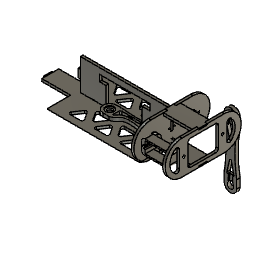
ERA v2.f3d (Autodesk Fusion 360 design; units mm, degrees)
Autodesk Fusion 360 part; units mm, degrees
(part 1 of 2)
sketch "Sketch1" plane through (0, 0, 0) normal (0, 0, 1) x (1, 0, 0)
  line L0 (0, 0) -> (22.8, 0)
  line L1 (22.8, 0) -> (22.8, 28.5)
  line L2 (22.8, 28.5) -> (0, 28.5)
  line L3 (0, 28.5) -> (0, 0)
  dimension "d1" = 22.8
  dimension "d2" = 28.5
  constraint horizontal L0
  constraint vertical L1
  constraint horizontal L2
  constraint vertical L3
  constraint coincident L0.start L3.end
  measures "d1" distance of L0.start L0.end
  measures "d2" distance of L0.start L2.end
sketch "Sketch2" plane through (0, 0, 0) normal (0, 0, 1) x (1, 0, 0)
  line L0 (-2.9, 21.5) -> (-1.5, 21.5)
  line L1 (-1.5, 21.5) -> (-1.5, 19)
  line L2 (-1.5, 19) -> (-2.9, 19)
  line L3 (-2.9, 19) -> (-2.9, 21.5)
  line L4 (0.5, 21.5) -> (1, 21.5)
  line L5 (1, 21.5) -> (1, 23)
  line L6 (1, 23) -> (0.5, 23)
  line L7 (0.5, 23) -> (0.5, 21.5)
  line L8 (-4.7224, 19.0074) -> (27.8871, 19.0074)
  line L9 (27.8871, 19.0074) -> (27.8871, 21.5074)
  line L10 (27.8871, 21.5074) -> (-4.7224, 21.5074)
  line L11 (-4.7224, 21.5074) -> (-4.7224, 19.0074)
  constraint horizontal L0
  constraint vertical L1
  constraint horizontal L2
  constraint vertical L3
  constraint horizontal L4
  constraint vertical L5
  constraint horizontal L6
  constraint vertical L7
  constraint horizontal L8
  constraint vertical L9
  constraint horizontal L10
  constraint vertical L11
sketch "Sketch3" plane through (0, 0, 0) normal (0, 0, 1) x (1, 0, 0)
  line L0 (0, 19) -> (18.5, 19)
  line L1 (18.5, 19) -> (18.5, 21)
  line L2 (18.5, 21) -> (0, 21)
  line L3 (0, 21) -> (0, 19)
  constraint horizontal L0
  constraint vertical L1
  constraint horizontal L2
  constraint vertical L3
sketch "Sketch4" plane through (0, 0, 0) normal (0, 0, 1) x (1, 0, 0)
  line L0 (-25, 0) -> (-47.8, 0)
  line L1 (-47.8, 0) -> (-47.8, 12.2)
  line L2 (-47.8, 12.2) -> (-25, 12.2)
  line L3 (-25, 12.2) -> (-25, 0)
  dimension "d3" = 22.8
  dimension "d4" = 12.2
  constraint horizontal L0
  constraint vertical L1
  constraint horizontal L2
  constraint vertical L3
  measures "d3" distance of L0.start L0.end
  measures "d4" distance of L0.start L2.end
extrude "Extrude1" add sketch "Sketch4" along normal blind 19 makes body 1
sketch "Sketch5" plane through (0, 0, 19) normal (0, 0, 1) x (-1, 0, 0)
  line L0 (25, -12.2) -> (47.8, -12.2)
  line L1 (47.8, -12.2) -> (47.8, 0)
  line L2 (47.8, 0) -> (25, 0)
  line L3 (25, 0) -> (25, -12.2)
  line L4 (52.7, 0) -> (20.1, 0)
  line L5 (20.1, 0) -> (20.1, -12.2)
  line L6 (20.1, -12.2) -> (52.7, -12.2)
  line L7 (52.7, -12.2) -> (52.7, 0)
  dimension "d7" = 32.6
  dimension "d8" = 12.2
  constraint horizontal L4
  constraint vertical L5
  constraint horizontal L6
  constraint vertical L7
  measures "d7" distance of L4.start L4.end
  measures "d8" distance of L4.start L6.end
extrude "Extrude2" add sketch "Sketch5" along normal blind 2.5 bodies 1
move_body "Move1" bodies 1 to x (1, 0, 0) y (0, 1, 0) z (0, 0, 1) at (0, 0, -21.5)
extrude "Extrude3" add sketch "Sketch4" along normal blind 1.5 bodies 1
sketch "Sketch6" plane through (0, 0, 1.5) normal (0, 0, 1) x (-1, 0, 0)
  line L0 (25, -12.2) -> (47.8, -12.2)
  line L1 (47.8, -12.2) -> (47.8, 0)
  line L2 (47.8, 0) -> (25, 0)
  line L3 (25, 0) -> (25, -12.2)
  circle A0 centre (31.1, -6.1) radius 6.1
  circle A1 centre (36.95, -6.05) radius 2
  dimension "d13" = 12.2
  dimension "d14" = 4
  measures "d13" diameter of A0
  measures "d14" diameter of A1
extrude "Extrude4" add sketch "Sketch6" along normal blind 5.5 contours A0 A1 | A0 A1 | A0 A1 bodies 1
sketch "Sketch7" plane through (0, 0, 7) normal (0, 0, 1) x (-1, 0, 0)
  arc A0 (36.8803, -8.0488) -> (36.8462, -4.0527) centre (36.95, -6.05) ccw
  arc A1 (36.8462, -4.0527) -> (36.8803, -8.0488) centre (31.1, -6.1) ccw
  circle A2 centre (31.1, -6.1) radius 2.5
  line L0 (31.1013, -8.6) -> (31.3, -8.3)
  line L1 (31.3, -8.3) -> (30.9, -8.3)
  line L2 (30.9, -8.3) -> (31.1013, -8.6)
  line L3 (31.296, -8.3004) -> (31.5477, -8.5596)
  line L4 (31.5477, -8.5596) -> (31.6896, -8.2289)
  line L5 (31.6858, -8.23) -> (31.9797, -8.4401)
  line L6 (31.9797, -8.4401) -> (32.0603, -8.0894)
  line L7 (32.0567, -8.0912) -> (32.3834, -8.2454)
  line L8 (32.3834, -8.2454) -> (32.4001, -7.886)
  line L9 (32.3969, -7.8883) -> (32.7459, -7.9818)
  line L10 (32.7459, -7.9818) -> (32.6981, -7.6252)
  line L11 (32.6953, -7.628) -> (33.0554, -7.6577)
  line L12 (33.0554, -7.6577) -> (32.9447, -7.3153)
  line L13 (32.9425, -7.3186) -> (33.3021, -7.2835)
  line L14 (33.3021, -7.2835) -> (33.1321, -6.9664)
  line L15 (33.1305, -6.97) -> (33.4781, -6.8713)
  line L16 (33.4781, -6.8713) -> (33.2541, -6.5896)
  line L17 (33.2532, -6.5935) -> (33.5776, -6.4343)
  line L18 (33.5776, -6.4343) -> (33.3069, -6.1971)
  line L19 (33.3068, -6.2011) -> (33.5974, -5.9865)
  line L20 (33.5974, -5.9865) -> (33.2888, -5.8015)
  line L21 (33.2893, -5.8054) -> (33.537, -5.5424)
  line L22 (33.537, -5.5424) -> (33.2003, -5.4155)
  line L23 (33.2016, -5.4193) -> (33.3983, -5.1162)
  line L24 (33.3983, -5.1162) -> (33.0444, -5.0514)
  line L25 (33.0462, -5.0549) -> (33.1857, -4.7216)
  line L26 (33.1857, -4.7216) -> (32.8259, -4.7211)
  line L27 (32.8284, -4.7242) -> (32.9061, -4.3714)
  line L28 (32.9061, -4.3714) -> (32.5519, -4.4351)
  line L29 (32.5549, -4.4377) -> (32.5684, -4.0767)
  line L30 (32.5684, -4.0767) -> (32.2313, -4.2026)
  line L31 (32.2347, -4.2046) -> (32.1835, -3.847)
  line L32 (32.1835, -3.847) -> (31.8743, -4.0311)
  line L33 (31.8781, -4.0325) -> (31.7638, -3.6897)
  line L34 (31.7638, -3.6897) -> (31.4925, -3.9261)
  line L35 (31.4964, -3.9268) -> (31.3228, -3.6099)
  line L36 (31.3228, -3.6099) -> (31.098, -3.8909)
  line L37 (31.102, -3.8909) -> (30.8746, -3.6102)
  line L38 (30.8746, -3.6102) -> (30.7036, -3.9268)
  line L39 (30.7075, -3.9261) -> (30.4336, -3.6904)
  line L40 (30.4336, -3.6904) -> (30.3219, -4.0325)
  line L41 (30.3256, -4.0311) -> (30.0141, -3.8482)
  line L42 (30.0141, -3.8482) -> (29.9653, -4.2046)
  line L43 (29.9687, -4.2026) -> (29.6295, -4.0782)
  line L44 (29.6295, -4.0782) -> (29.6451, -4.4377)
  line L45 (29.6481, -4.4351) -> (29.2921, -4.3733)
  line L46 (29.2921, -4.3733) -> (29.3716, -4.7242)
  line L47 (29.3741, -4.7211) -> (29.0128, -4.7239)
  line L48 (29.0128, -4.7239) -> (29.1538, -5.0549)
  line L49 (29.1556, -5.0514) -> (28.8007, -5.1187)
  line L50 (28.8007, -5.1187) -> (28.9984, -5.4193)
  line L51 (28.9997, -5.4155) -> (28.6624, -5.545)
  line L52 (28.6624, -5.545) -> (28.9107, -5.8054)
  line L53 (28.9112, -5.8015) -> (28.6025, -5.9892)
  line L54 (28.6025, -5.9892) -> (28.8932, -6.2011)
  line L55 (28.8931, -6.1971) -> (28.6228, -6.4369)
  line L56 (28.6228, -6.4369) -> (28.9468, -6.5935)
  line L57 (28.9459, -6.5896) -> (28.7228, -6.8738)
  line L58 (28.7228, -6.8738) -> (29.0695, -6.97)
  line L59 (29.0679, -6.9664) -> (28.8991, -7.2858)
  line L60 (28.8991, -7.2858) -> (29.2575, -7.3186)
  line L61 (29.2553, -7.3153) -> (29.1463, -7.6598)
  line L62 (29.1463, -7.6598) -> (29.5047, -7.628)
  line L63 (29.5019, -7.6252) -> (29.4562, -7.9836)
  line L64 (29.4562, -7.9836) -> (29.8031, -7.8883)
  line L65 (29.7999, -7.886) -> (29.8189, -8.2468)
  line L66 (29.8189, -8.2468) -> (30.1433, -8.0912)
  line L67 (30.1397, -8.0894) -> (30.2228, -8.4411)
  line L68 (30.2228, -8.4411) -> (30.5142, -8.23)
  line L69 (30.5104, -8.2289) -> (30.6549, -8.5601)
  line L70 (30.6549, -8.5601) -> (30.904, -8.3004)
  dimension "d17" = 5
  dimension "d19" = 360
  constraint concentric A1 A2
  constraint coincident A2 L0.start
  constraint horizontal L1
  measures "d17" diameter of A2
extrude "Extrude5" add sketch "Sketch7" along normal blind 4 contours L0 L1 L2 L3 L4 L5 L6 L7 L8 L9 L10 L11 L12 L13 L14 L15 L16 L17 L18 L19 L20 L21 L22 L23 L24 L25 L26 L27 L28 L29 L30 L31 L32 L33 L34 L35 L36 L37 L38 L39 L40 L41 L42 L43 L44 L45 L46 L47 L48 L49 L50 L51 L52 L53 L54 L55 L56 L57 L58 L59 L60 L61 L62 L63 L64 L65 L66 L67 L68 L69 L70 | L0 L1 L2 L3 L70 | L0 L1 L3 | L1 L2 L70 bodies 1
move_body "Move2" bodies 1 to x (1, 0, 0) y (0, 1, 0) z (0, 0, 1) at (0, 0, 21.5)
sketch "Sketch8" plane through (0, 0, 0) normal (0, 0, 1) x (1, 0, 0)
  line L0 (0, 0) -> (77.5, 0)
  line L1 (77.5, 0) -> (77.5, 41.5)
  line L2 (77.5, 41.5) -> (0, 41.5)
  line L3 (0, 41.5) -> (0, 0)
  line L4 (0, 0) -> (77.5, 0)
  line L5 (77.5, 0) -> (77.5, 1)
  line L6 (77.5, 1) -> (0, 1)
  line L7 (0, 1) -> (0, 0)
  line L8 (77.5, 0) -> (76.5, 0)
  line L9 (76.5, 0) -> (76.5, 41.5)
  line L10 (76.5, 41.5) -> (77.5, 41.5)
  line L11 (77.5, 41.5) -> (77.5, 0)
  line L12 (0, 41.5) -> (77.5, 41.5)
  line L13 (77.5, 41.5) -> (77.5, 40.5)
  line L14 (77.5, 40.5) -> (0, 40.5)
  line L15 (0, 40.5) -> (0, 41.5)
  line L16 (0, 41.5) -> (1, 41.5)
  line L17 (1, 41.5) -> (1, 0)
  line L18 (1, 0) -> (0, 0)
  line L19 (0, 0) -> (0, 41.5)
  line L20 (0, 22) -> (77.5, 22)
  line L21 (77.5, 22) -> (77.5, 20)
  line L22 (77.5, 20) -> (0, 20)
  line L23 (0, 20) -> (0, 22)
  dimension "d22" = 77.5
  dimension "d23" = 41.5
  dimension "d24" = 1
  dimension "d25" = 1
  dimension "d26" = 1
  dimension "d27" = 1
  dimension "d28" = 41.5
  dimension "d29" = 77.5
  dimension "d30" = 2
  constraint horizontal L0
  constraint vertical L1
  constraint horizontal L2
  constraint vertical L3
  constraint coincident L0.start L3.end
  constraint horizontal L4
  constraint vertical L5
  constraint horizontal L6
  constraint vertical L7
  constraint horizontal L8
  constraint vertical L9
  constraint horizontal L10
  constraint vertical L11
  constraint coincident L2 L9.end
  constraint horizontal L12
  constraint vertical L13
  constraint horizontal L14
  constraint vertical L15
  constraint coincident L11 L13.end
  constraint horizontal L16
  constraint vertical L17
  constraint horizontal L18
  constraint vertical L19
  constraint horizontal L20
  constraint vertical L21
  constraint horizontal L22
  constraint vertical L23
  constraint coincident L19 L20.start
  measures "d22" distance of L0.start L0.end
  measures "d23" distance of L0.start L2.end
  measures "d24" distance of L0.start L6.end
  measures "d25" distance of L0.end L8.end
  measures "d26" distance of L2.end L14.end
  measures "d27" distance of L2.end L16.end
  measures "d28" distance of L2.end L0.start
  measures "d29" distance of L20.start L20.end
  measures "d30" distance of L20.start L22.end
extrude "Extrude6" add sketch "Sketch8" along normal blind 21.5 separate body contours L0 L3 L4 L6 L7 L17 L18 L19 | L3 L6 L17 L19 L22 | L0 L1 L4 L5 L6 L8 L9 L11 | L3 L17 L19 L20 L22 L23 | L1 L6 L9 L11 L22 | L3 L14 L17 L19 L20 | L1 L9 L11 L20 L21 L22 | L2 L3 L12 L14 L15 L16 L17 L19 | L1 L9 L11 L14 L20 | L1 L2 L9 L10 L11 L12 L13 L14 makes body 2 at (0, 27.6667, 14.3333) makes body 3 at (76.5, 13.8333, 14.3333)
extrude "Extrude7" add sketch "Sketch8" along normal blind 10 contours L0 L4 L6 L9 L17 | L9 L17 L20 L22 | L2 L9 L12 L14 L17 bodies 2 3
extrude "Extrude8" add sketch "Sketch8" along normal blind 1 contours L6 L9 L17 L22 | L9 L14 L17 L20 bodies 2
fillet "Fillet1" radius 5 4 edges at (38.75, 40.5, 1) (38.75, 20, 1) (38.75, 1, 1) (38.75, 22, 1) on bodies 2
fillet "Fillet2" radius 5 6 edges at (1, 0.5, 10) (1, 21, 10) (1, 41, 10) (76.5, 41, 10) (76.5, 21, 10) (76.5, 0.5, 10) on bodies 2
move_body "Move3" bodies 1 to x (1, 0, 0) y (0, 0, 1) z (0, -1, 0) at (0, 0, 0)
copy_body "CopyPasteBodies1" bodies 1 makes body 4
move_body "Move4" bodies 4 to x (1, 0, 0) y (0, -1, 0) z (0, 0, -1) at (0, 41.5, 12)
copy_body "CopyPasteBodies2" bodies 4 1 makes body 5 makes body 6
move_body "Move5" bodies 5 6 to x (1, 0, 0) y (0, 1, 0) z (0, 0, 1) at (150, 0, 0)
sketch "Sketch9" plane through (0, 0, 1) normal (0, 0, 1) x (-1, 0, 0)
  line L0 (-1, -6) -> (-76.5, -6)
  line L1 (-76.5, -6) -> (-76.5, -15)
  line L2 (-76.5, -15) -> (-1, -15)
  line L3 (-1, -15) -> (-1, -6)
  line L4 (144.7876, -93.3118) -> (-10.828, -93.3118) construction
  line L5 (-10.828, -93.3118) -> (-10.828, -128.7007) construction
  line L6 (-10.828, -128.7007) -> (144.7876, -128.7007) construction
  line L7 (144.7876, -128.7007) -> (144.7876, -93.3118) construction
move_body "Move6" bodies 1 4 to x (-1, 0, 0) y (0, 1, 0) z (0, 0, -1) at (-75.4, 0, 12)
move_body "Move7" bodies 1 to x (0, 1, 0) y (1, 0, 0) z (0, 0, -1) at (-27.5, 27.5, 12)
move_body "Move8" bodies 4 to x (0, -1, 0) y (-1, 0, 0) z (0, 0, -1) at (14, 14, 12.4)
move_body "Move9" bodies 5 to x (0, 1, 0) y (1, 0, 0) z (0, 0, -1) at (60.6, -60.6, 12)
move_body "Move10" bodies 6 to x (0, -1, 0) y (-1, 0, 0) z (0, 0, -1) at (102.1, 102.1, 12.4)
move_body "Move11" bodies 1 4 to x (1, 0, 0) y (0, 1, 0) z (0, 0, 1) at (25, 0, 0)
move_body "Move12" bodies 5 6 to x (1, 0, 0) y (0, 1, 0) z (0, 0, 1) at (-22, 0, 0)
move_body "Move13" bodies 1 6 to x (1, 0, 0) y (0, 1, 0) z (0, 0, 1) at (0, 16, 0)
move_body "Move14" bodies 4 5 to x (1, 0, 0) y (0, 1, 0) z (0, 0, 1) at (0, -13, 0)
move_body "Move15" bodies 2 to x (1, 0, 0) y (0, 1, 0) z (0, 0, 1) at (0, -1, 0)
move_body "Move16" bodies 1 6 to x (1, 0, 0) y (0, 1, 0) z (0, 0, 1) at (0, -5.8, 0)
move_body "Move17" bodies 4 5 to x (1, 0, 0) y (0, 1, 0) z (0, 0, 1) at (0, 1.3, 0)
copy_body "CopyPasteBodies3" bodies 1 4 5 6 makes body 7 makes body 8 makes body 9 makes body 10
move_body "Move18" bodies 7 8 9 10 to x (1, 0, 0) y (0, 1, 0) z (0, 0, 1) at (0, -130, 0)
move_body "Move19" bodies 7 to x (0, -1, 0) y (1, 0, 0) z (0, 0, 1) at (80, 29.7, 0)
move_body "Move20" bodies 8 to x (0, 1, 0) y (-1, 0, 0) z (0, 0, 1) at (-139.7, 10.3, 0)
move_body "Move21" bodies 10 to x (0, 1, 0) y (-1, 0, 0) z (0, 0, 1) at (-2.7, -47.9, 0)
move_body "Move22" bodies 9 to x (0, -1, 0) y (1, 0, 0) z (0, 0, 1) at (217.3, 87.9, 0)
move_body "Move23" bodies 1 6 8 9 to x (1, 0, 0) y (0, 1, 0) z (0, 0, 1) at (0, -0.8, 0)
move_body "Move24" bodies 4 5 7 10 to x (1, 0, 0) y (0, 1, 0) z (0, 0, 1) at (0, 0.8, 0)
move_body "Move25" bodies 1 6 8 9 to x (1, 0, 0) y (0, 1, 0) z (0, 0, 1) at (0, -4.5, 0)
move_body "Move26" bodies 4 5 7 10 to x (1, 0, 0) y (0, 1, 0) z (0, 0, 1) at (0, 4.5, 0)
move_body "Move27" bodies 2 to x (1, 0, 0) y (0, 1, 0) z (0, 0, 1) at (0, 170, 0)
move_body "Move28" bodies 5 6 10 9 to x (1, 0, 0) y (0, 1, 0) z (0, 0, 1) at (-34.956, 0, 0)
move_body "Move29" bodies 2 to x (0, 1, 0) y (-1, 0, 0) z (0, 0, 1) at (208, -18.75, 0)
move_body "Move30" bodies 5 6 10 9 to x (1, 0, 0) y (0, 1, 0) z (0, 0, 1) at (-6, 0, 0)
move_body "Move31" bodies 5 6 10 9 to x (1, 0, 0) y (0, 1, 0) z (0, 0, 1) at (5.75, 0, 0)
move_body "Move32" bodies 2 to x (1, 0, 0) y (0, 1, 0) z (0, 0, 1) at (3, 0, 0)
sketch "Sketch10" plane through (0, 0, 0) normal (0, 0, 1) x (1, 0, 0)
  line L0 (-80, -30) -> (120, -30)
  line L1 (120, -30) -> (120, 60)
  line L2 (120, 60) -> (-80, 60)
  line L3 (-80, 60) -> (-80, -30)
  dimension "d41" = 200
  dimension "d42" = 90
  constraint horizontal L0
  constraint vertical L1
  constraint horizontal L2
  constraint vertical L3
  measures "d41" distance of L0.start L0.end
  measures "d42" distance of L0.start L2.end
move_body "Move33" bodies 2 9 4 5 6 1 7 10 8 to x (1, 0, 0) y (0, 1, 0) z (0, 0, 1) at (-1, -5, 0)
move_body "Move34" bodies 2 9 4 5 6 1 7 10 8 to x (1, 0, 0) y (0, 1, 0) z (0, 0, 1) at (0, 0, 4)
move_body "Move35" bodies 4 5 to x (1, 0, 0) y (0, 1, 0) z (0, 0, 1) at (0, -10, 0)
move_body "Move36" bodies 1 6 to x (1, 0, 0) y (0, 1, 0) z (0, 0, 1) at (0, 10, 0)
move_body "Move37" bodies 4 1 to x (1, 0, 0) y (0, 1, 0) z (0, 0, 1) at (-3, 0, 0)
move_body "Move38" bodies 5 6 to x (1, 0, 0) y (0, 1, 0) z (0, 0, 1) at (3, 0, 0)
sketch "Sketch11" plane through (0, 0, 4) normal (0, 0, 1) x (-1, 0, 0)
  line L0 (80, -60) -> (80, 30)
  line L1 (80, 30) -> (-120, 30)
  line L2 (-120, 30) -> (-120, -60)
  line L3 (-120, -60) -> (80, -60)
  line L4 (80, -60) -> (-120, -60)
  line L5 (-120, -60) -> (-120, -56)
  line L6 (-120, -56) -> (80, -56)
  line L7 (80, -56) -> (80, -60)
  line L8 (80, -60) -> (76, -60)
  line L9 (76, -60) -> (76, 30)
  line L10 (76, 30) -> (80, 30)
  line L11 (80, 30) -> (80, -60)
  line L12 (80, 30) -> (-120, 30)
  line L13 (-120, 30) -> (-120, 26)
  line L14 (-120, 26) -> (80, 26)
  line L15 (80, 26) -> (80, 30)
  line L16 (-120, -60) -> (-116, -60)
  line L17 (-116, -60) -> (-116, 30)
  line L18 (-116, 30) -> (-120, 30)
  line L19 (-120, 30) -> (-120, -60)
  dimension "d47" = 4
  dimension "d48" = 4
  dimension "d49" = 4
  dimension "d50" = 4
  constraint horizontal L4
  constraint vertical L5
  constraint horizontal L6
  constraint vertical L7
  constraint coincident L0.start L3.end
  constraint horizontal L8
  constraint vertical L9
  constraint horizontal L10
  constraint vertical L11
  constraint horizontal L12
  constraint vertical L13
  constraint horizontal L14
  constraint vertical L15
  constraint horizontal L16
  constraint vertical L17
  constraint horizontal L18
  constraint vertical L19
  measures "d47" distance of L0.start L6.end
  measures "d48" distance of L0.start L8.end
  measures "d49" distance of L0.end L14.end
  measures "d50" distance of L2.end L16.end
sketch "Sketch12" plane through (-25.5, 0, 0) normal (1, 0, 0) x (0, 1, 0)
  line L0 (-13, 4) -> (-13, 16.2)
  line L1 (-13, 16.2) -> (-17.9, 16.2)
  line L2 (-17.9, 16.2) -> (-17.9, 4)
  line L3 (-17.9, 4) -> (-13, 4)
  line L4 (-13.6, 3.4) -> (10.4, 3.4)
  line L5 (10.4, 3.4) -> (10.4, 16.8)
  line L6 (10.4, 16.8) -> (-13.6, 16.8)
  line L7 (-13.6, 16.8) -> (-13.6, 3.4)
  line L8 (-17.9, 1.6) -> (14.7, 1.6)
  line L9 (14.7, 1.6) -> (14.7, 18.6)
  line L10 (14.7, 18.6) -> (-17.9, 18.6)
  line L11 (-17.9, 18.6) -> (-17.9, 1.6)
  circle A0 centre (-15.9807, 10.1) radius 1
  circle A1 centre (13.0442, 10.1) radius 1
  dimension "d58" = 24
  dimension "d59" = 13.4
  dimension "d60" = 32.6
  dimension "d61" = 17
  dimension "d62" = 2
  dimension "d63" = 2
  constraint horizontal L4
  constraint vertical L5
  constraint horizontal L6
  constraint vertical L7
  constraint horizontal L8
  constraint vertical L9
  constraint horizontal L10
  constraint vertical L11
  measures "d58" distance of L4.start L4.end
  measures "d59" distance of L4.start L6.end
  measures "d60" distance of L8.start L8.end
  measures "d61" distance of L8.start L10.end
  measures "d62" diameter of A0
  measures "d63" diameter of A1
extrude "Extrude11" add sketch "Sketch12" along normal blind 10 separate body contours L1 L3 L4 L5 L6 L7 L8 L9 L10 L11 | L1 L2 L3 L7 L11 makes body 11
sketch "Sketch13" plane through (0, 14.7, 0) normal (0, 1, 0) x (-1, 0, 0)
  line L0 (25.5, 1.6) -> (25.5, 18.6)
  line L1 (25.5, 18.6) -> (15.5, 18.6)
  line L2 (15.5, 18.6) -> (15.5, 1.6)
  line L3 (15.5, 1.6) -> (25.5, 1.6)
  line L4 (25.5, 18.6) -> (6.5, 18.6)
  line L5 (6.5, 18.6) -> (6.5, 1.6)
  line L6 (6.5, 1.6) -> (25.5, 1.6)
  line L7 (25.5, 1.6) -> (25.5, 18.6)
  circle A0 centre (12, 10.1) radius 3.5
  line L8 (15.5, 18.6) -> (15.5, 17.6)
  line L9 (15.5, 1.6) -> (15.5, 2.6)
  line L10 (15.5, 17.6) -> (6.5, 14.5586)
  line L11 (15.5, 2.6) -> (6.5, 5.6414)
  dimension "d66" = 19
  dimension "d67" = 17
  dimension "d68" = 7
  dimension "d69" = 1
  dimension "d70" = 1
  dimension "d107" = 9.5
  dimension "d108" = 9.5
  constraint horizontal L4
  constraint vertical L5
  constraint horizontal L6
  constraint vertical L7
  constraint coincident L0.end L1.start
  constraint coincident L1.end L2.start
  constraint coincident L2 L8.end
  constraint coincident L2.end L3.start
  constraint perpendicular L6 L9
  constraint coincident L5 L10.end
  constraint coincident L5 L11.end
  measures "d66" distance of L0.end L4.end
  measures "d67" distance of L0.end L0.start
  measures "d68" diameter of A0
  measures "d69" distance of L1.end L8.end
  measures "d70" distance of L2.end L9.end
  measures "d107" distance of L8.end L10.end
  measures "d108" distance of L9.end L11.end
extrude "Extrude12" add sketch "Sketch13" against normal blind 4.3 contours L2 L5 L10 L11 bodies 11
sketch "Sketch14" plane through (0, 10.4, 0) normal (0, -1, 0) x (1, 0, 0)
  circle A0 centre (-12, 10.1) radius 3.5
  line L0 (-6.5, 5.6414) -> (-6.5, 14.5586)
  line L1 (-15.5, 3.4) -> (-15.5, 2.6)
  line L2 (-15.5, 16.8) -> (-25.5, 16.8)
  line L3 (-25.5, 16.8) -> (-25.5, 3.4)
  line L4 (-25.5, 3.4) -> (-15.5, 3.4)
  line L5 (-25.5146, 12.3255) -> (-25.5146, 7.9255)
  line L6 (-25.5146, 12.3255) -> (-14.0316, 12.95)
  line L7 (-14.0316, 12.95) -> (-14.0316, 7.25)
  line L8 (-14.0316, 7.25) -> (-25.5146, 7.9255)
  line L9 (-15.5, 2.6) -> (-6.5, 5.6414)
  line L10 (-6.5, 14.5586) -> (-15.5, 17.6)
  line L11 (-15.5, 17.6) -> (-15.5, 16.8)
  dimension "d79" = 4.4
  dimension "d81" = 11.5
  dimension "d82" = 5.7
  constraint vertical L5
  constraint coincident A0 L6.end
  measures "d79" distance of L5.start L5.end
  measures "d81" distance of L5.start L6.end
  measures "d82" distance of L6.end L7.end
extrude "Extrude13" cut sketch "Sketch14" against normal blind 2 contours A0 L3 L6 L8 bodies 11
sketch "Sketch15" plane through (0, -17.9, 0) normal (0, -1, 0) x (1, 0, 0)
  line L0 (-15.5, 1.6) -> (-15.5, 18.6)
  line L1 (-25.5, 18.6) -> (-25.5, 1.6)
  circle A0 centre (-12, 10.1) radius 1.5
  line L2 (-15.5, 18.6) -> (-10.5, 18.6) construction
  line L3 (-15.5, 1.6) -> (-10.5, 1.6) construction
  line L4 (-25.5, 1.6) -> (-15.5, 1.6)
  line L5 (-15.5, 18.6) -> (-25.5, 18.6)
  line L6 (-15.5, 18.6) -> (-8.5, 18.6)
  line L7 (-8.5, 18.6) -> (-8.5, 1.6)
  line L8 (-8.5, 1.6) -> (-15.5, 1.6)
  line L9 (-15.5, 1.6) -> (-15.5, 18.6)
  line L10 (-15.5, 18.6) -> (-15.4999, 18.6)
  line L11 (-15.4999, 18.6) -> (-15.4999, 16.6)
  line L12 (-15.4999, 16.6) -> (-15.5, 16.6)
  line L13 (-15.5, 16.6) -> (-15.5, 18.6)
  line L14 (-15.5, 1.6) -> (-15.5, 3.6)
  line L15 (-15.5, 3.6) -> (-8.5, 8.4218)
  line L16 (-15.4999, 16.6) -> (-8.5, 11.778)
  dimension "d86" = 3
  dimension "d97" = 7
  dimension "d98" = 17
  dimension "d99" = 2
  dimension "d100" = 2
  dimension "d101" = 8.5
  dimension "d102" = 8.5
  constraint horizontal L2
  constraint coincident L0.end L2.start
  constraint horizontal L3
  constraint coincident L0.start L3.start
  constraint horizontal L6
  constraint vertical L7
  constraint horizontal L8
  constraint vertical L9
  constraint horizontal L10
  constraint vertical L11
  constraint horizontal L12
  constraint vertical L13
  constraint perpendicular L8 L14
  constraint coincident L7 L15.end
  constraint coincident L7 L16.end
  measures "d86" diameter of A0
  measures "d97" distance of L0.end L6.end
  measures "d98" distance of L0.end L0.start
  measures "d99" distance of L0.end L12.end
  measures "d100" distance of L0.start L14.end
  measures "d101" distance of L14.end L15.end
  measures "d102" distance of L11.end L16.end
extrude "Extrude14" add sketch "Sketch15" against normal blind 4.3 contours L0 L7 L9 L15 L16 bodies 11
fillet "Fillet9" radius 3 2 edges at (-8.5, -15.75, 11.778) (-8.5, -15.75, 8.4218) on bodies 11
fillet "Fillet10" radius 4 4 edges at (-20.5, -17.9, 18.6) (-20.5, 14.7, 18.6) (-20.5, -17.9, 1.6) (-20.5, 14.7, 1.6) on bodies 11
fillet "Fillet11" radius 4 2 edges at (-6.5, 12.55, 14.5586) (-6.5, 12.55, 5.6414) on bodies 11
move_body "Move39" bodies 11 to x (0, 1, 0) y (1, 0, 0) z (0, 0, -1) at (-50.6, 4.1, 20.2)
copy_body "CopyPasteBodies4" bodies 11 makes body 12
move_body "Move40" bodies 12 to x (1, 0, 0) y (0, 1, 0) z (0, 0, 1) at (-40, 0, 0)
copy_body "CopyPasteBodies5" bodies 11 makes body 13
move_body "Move41" bodies 13 to x (1, 0, 0) y (0, 1, 0) z (0, 0, 1) at (-80, 0, 0)
copy_body "CopyPasteBodies6" bodies 11 makes body 14
move_body "Move42" bodies 14 to x (1, 0, 0) y (0, 1, 0) z (0, 0, 1) at (-120, 0, 0)
move_body "Move43" bodies 12 to x (1, 0, 0) y (0, -1, 0) z (0, 0, -1) at (40, 30.1, 20.2)
move_body "Move44" bodies 13 to x (-1, 0, 0) y (0, -1, 0) z (0, 0, 1) at (-40, 30.1, 0)
move_body "Move45" bodies 14 to x (-1, 0, 0) y (0, 1, 0) z (0, 0, -1) at (-80, 0, 20.2)
sketch "Sketch16" plane through (108.5, 0, 0) normal (1, 0, 0) x (0, 1, 0)
  line L0 (-21.4, 5.6) -> (-8.4965, 5.6)
  line L1 (-8.4965, 5.6) -> (-5.6982, 7.5276)
  arc A0 (-5.6982, 7.5276) -> (-4.4, 9.9982) centre (-7.4, 9.9982) ccw
  line L2 (-4.4, 9.9982) -> (-4.4, 10.2017)
  arc A1 (-4.4, 10.2017) -> (-5.6981, 12.6723) centre (-7.4, 10.2017) ccw
  line L3 (-5.6981, 12.6723) -> (-8.4966, 14.6)
  line L4 (-8.4966, 14.6) -> (-21.4, 14.6)
  line L5 (-21.4, 14.6) -> (-21.4, 5.6)
  circle A2 centre (-7.9, 10.1) radius 1.5
  line L6 (-30, 0) -> (60, 0)
  line L7 (60, 0) -> (60, 40)
  line L8 (60, 40) -> (-30, 40)
  line L9 (-30, 40) -> (-30, 0)
  circle A3 centre (-8.0417, 20.0231) radius 1.5
  line L10 (-8.0417, 20.0231) -> (37.9583, 20.0231)
  circle A4 centre (37.9583, 20.0231) radius 1.5
  dimension "d111" = 90
  dimension "d112" = 40
  dimension "d113" = 3
  dimension "d115" = 46
  dimension "d116" = 3
  constraint horizontal L6
  constraint vertical L7
  constraint horizontal L8
  constraint vertical L9
  constraint coincident A3.centre L10.start
  constraint horizontal L10
  constraint coincident L10.end A4.centre
  measures "d111" distance of L6.start L6.end
  measures "d112" distance of L6.start L8.end
  measures "d113" diameter of A3
  measures "d115" distance of A3.centre L10.end
  measures "d116" diameter of A4
extrude "Extrude15" add sketch "Sketch16" along normal blind 3 separate body contours L0 L1 A0 L2 A1 L3 L4 L5 | A2 | L6 L7 L8 L9 makes body 15
fillet "Fillet12" radius 20 4 edges at (110, -30, 40) (110, -30, 0) (110, 60, 0) (110, 60, 40) on bodies 15
sketch "Sketch17" plane through (111.5, 0, 0) normal (1, 0, 0) x (0, 1, 0)
  arc A0 (40, 0) -> (40, 40) centre (40, 20) ccw
  line L0 (40, 40) -> (-10, 40)
  arc A1 (-10, 40) -> (-10, 0) centre (-10, 20) ccw
  line L1 (-10, 0) -> (40, 0)
  circle A2 centre (-8.0417, 20.0231) radius 1.5
  circle A3 centre (37.9583, 20.0231) radius 1.5
  line L2 (-3, 35) -> (33, 35)
  line L3 (33, 35) -> (33, 5)
  line L4 (33, 5) -> (-3, 5)
  line L5 (-3, 5) -> (-3, 35)
  line L6 (-30, 20) -> (-24.3622, 20)
  line L7 (60, 20) -> (52.8569, 20)
  line L8 (43, 35) -> (43, 5)
  line L9 (-13, 35) -> (-13, 5)
  arc A4 (-13, 35) -> (-13, 5) centre (-8.7798, 20) ccw
  arc A5 (43, 5) -> (43, 35) centre (36.5151, 20) ccw
  dimension "d121" = 36
  dimension "d122" = 30
  constraint horizontal L2
  constraint vertical L3
  constraint horizontal L4
  constraint vertical L5
  constraint midpoint A1 L6.start
  constraint horizontal L6
  constraint midpoint A0 L7.start
  constraint perpendicular L2 L8
  constraint vertical L9
  constraint coincident L6.end A4
  constraint coincident L7.end A5
  measures "d121" distance of L2.start L2.end
  measures "d122" distance of L2.start L4.end
extrude "Extrude16" cut sketch "Sketch17" against normal blind 4 contours L2 L3 L4 L5 | L8 A5 | L9 A4 bodies 15
fillet "Fillet13" radius 3 8 edges at (110, 33, 35) (110, -3, 35) (110, 33, 5) (110, -3, 5) (110, -13, 5) (110, -13, 35) (110, 43, 35) (110, 43, 5) on bodies 15
sketch "Sketch18" plane through (0, 0, 40) normal (0, 0, 1) x (-1, 0, 0)
  line L0 (-111.5, -40) -> (-108.5, -40)
  line L1 (-108.5, -40) -> (-108.5, 10)
  line L2 (-111.5, 10) -> (-111.5, -40)
  line L3 (-74.5, -25) -> (-108.5, -25)
  line L4 (-108.5, -25) -> (-108.5, -5)
  line L5 (-108.5, -5) -> (-74.5, -5)
  line L6 (-74.5, -5) -> (-74.5, -25)
  line L7 (-110, 15) -> (-110, -15)
  line L8 (-108.5, -20) -> (-111.5, -20)
  line L9 (-111.5, -20) -> (-111.5, -10)
  line L10 (-111.5, -10) -> (-108.5, -10)
  line L11 (-108.5, -10) -> (-108.5, -20)
  line L12 (-74.5, -15) -> (35.5, -15)
  line L13 (35.5, -15) -> (35.5, -53)
  line L14 (35.5, -53) -> (-74.5, -53)
  line L15 (-74.5, -53) -> (-74.5, -15)
  line L16 (-74.5, -15) -> (35.5, -15)
  line L17 (35.5, -15) -> (35.5, 23)
  line L18 (35.5, 23) -> (-74.5, 23)
  line L19 (-74.5, 23) -> (-74.5, -15)
  line L20 (35.5, -15) -> (69.5, -15)
  line L21 (69.5, -15) -> (69.5, -25)
  line L22 (69.5, -25) -> (35.5, -25)
  line L23 (35.5, -25) -> (35.5, -15)
  line L24 (35.5, -15) -> (69.5, -15)
  line L25 (69.5, -15) -> (69.5, -5)
  line L26 (69.5, -5) -> (35.5, -5)
  line L27 (35.5, -5) -> (35.5, -15)
  line L28 (69.5, -15) -> (72.5, -15)
  line L29 (72.5, -15) -> (72.5, -20)
  line L30 (72.5, -20) -> (69.5, -20)
  line L31 (69.5, -20) -> (69.5, -15)
  line L32 (69.5, -15) -> (72.5, -15)
  line L33 (72.5, -15) -> (72.5, -10)
  line L34 (72.5, -10) -> (69.5, -10)
  line L35 (69.5, -10) -> (69.5, -15)
  line L36 (-108.5, 10) -> (-111.5, 10)
  dimension "d127" = 34
  dimension "d128" = 20
  dimension "d129" = 30
  dimension "d130" = 3
  dimension "d131" = 10
  dimension "d132" = 110
  dimension "d133" = 38
  dimension "d134" = 38
  dimension "d135" = 34
  dimension "d136" = 10
  dimension "d137" = 10
  dimension "d138" = 3
  dimension "d139" = 5
  constraint horizontal L3
  constraint vertical L4
  constraint horizontal L5
  constraint vertical L6
  constraint coincident L1 L3.end
  constraint horizontal L8
  constraint vertical L9
  constraint horizontal L10
  constraint vertical L11
  constraint coincident L1 L8.start
  constraint horizontal L12
  constraint vertical L13
  constraint horizontal L14
  constraint vertical L15
  constraint midpoint L6 L12.start
  constraint horizontal L16
  constraint vertical L17
  constraint horizontal L18
  constraint vertical L19
  constraint horizontal L20
  constraint vertical L21
  constraint horizontal L22
  constraint vertical L23
  constraint horizontal L24
  constraint vertical L25
  constraint horizontal L26
  constraint vertical L27
  constraint horizontal L28
  constraint vertical L29
  constraint horizontal L30
  constraint vertical L31
  constraint horizontal L32
  constraint vertical L33
  constraint horizontal L34
  constraint vertical L35
  measures "d127" distance of L3.start L3.end
  measures "d128" distance of L3.start L5.end
  measures "d129" distance of L7.start L7.end
  measures "d130" distance of L8.start L8.end
  measures "d131" distance of L8.start L10.end
  measures "d132" distance of L12.start L12.end
  measures "d133" distance of L12.start L14.end
  measures "d134" distance of L12.start L18.end
  measures "d135" distance of L12.end L20.end
  measures "d136" distance of L12.end L22.end
  measures "d137" distance of L12.end L26.end
  measures "d138" distance of L20.end L28.end
  measures "d139" distance of L20.end L34.end
extrude "Extrude17" add sketch "Sketch18" along normal blind 3 separate body contours L1 L2 L4 L8 L9 L10 L11 | L1 L3 L4 L5 L6 L11 L15 L19 | L6 L12 L13 L14 L15 L16 L23 | L6 L12 L16 L17 L18 L19 L27 | L13 L20 L21 L22 L23 L24 L31 | L17 L20 L24 L25 L26 L27 L35 | L21 L28 L29 L30 L31 L32 | L25 L28 L32 L33 L34 L35 makes body 16
sketch "Sketch19" plane through (111.5, 0, 0) normal (1, 0, 0) x (0, 1, 0)
  line L0 (33, 32) -> (33, 8)
  line L1 (30, 5) -> (0, 5)
  line L2 (-3, 8) -> (-3, 32)
  line L3 (0, 35) -> (30, 35)
  arc A0 (40, 0) -> (40, 40) centre (40, 20) ccw
  line L4 (40, 40) -> (-10, 40)
  arc A1 (-10, 40) -> (-10, 0) centre (-10, 20) ccw
  line L5 (-10, 0) -> (40, 0)
  circle A2 centre (-8.0417, 20.0231) radius 1.5
  circle A3 centre (37.9583, 20.0231) radius 1.5
  line L6 (15, 40) -> (20, 40)
  line L7 (20, 40) -> (20, 38.5)
  line L8 (20, 38.5) -> (15, 38.5)
  line L9 (15, 38.5) -> (15, 40)
  line L10 (15, 40) -> (10, 40)
  line L11 (15, 38.4991) -> (15, 40)
  line L12 (15, 40) -> (10, 40)
  line L13 (10, 40) -> (10, 38.5)
  line L14 (10, 38.5) -> (15, 38.5)
  line L15 (15, 38.5) -> (15, 40)
  line L16 (10, 0) -> (20, 0)
  line L17 (20, 0) -> (20, 1.5)
  line L18 (20, 1.5) -> (10, 1.5)
  line L19 (10, 1.5) -> (10, 0)
  arc A4 (30, 5) -> (33, 8) centre (30, 8) ccw
  arc A5 (-3, 8) -> (0, 5) centre (0, 8) ccw
  arc A6 (0, 35) -> (-3, 32) centre (0, 32) ccw
  arc A7 (33, 32) -> (30, 35) centre (30, 32) ccw
  line L20 (-13, 30.3046) -> (-13, 9.6954)
  arc A8 (-17.7215, 32.7615) -> (-17.7215, 7.2385) centre (-8.7798, 20) ccw
  line L21 (43, 10.617) -> (43, 29.383)
  arc A9 (48.1328, 8.5072) -> (48.1328, 31.4928) centre (36.5151, 20) ccw
  arc A10 (-17.7215, 7.2385) -> (-13, 9.6954) centre (-16, 9.6954) ccw
  arc A11 (-13, 30.3046) -> (-17.7215, 32.7615) centre (-16, 30.3046) ccw
  arc A12 (48.1328, 31.4928) -> (43, 29.383) centre (46, 29.383) ccw
  arc A13 (43, 10.617) -> (48.1328, 8.5072) centre (46, 10.617) ccw
  dimension "d142" = 1.5
  dimension "d143" = 5
  dimension "d149" = 1.5
  constraint horizontal L6
  constraint vertical L7
  constraint horizontal L8
  constraint vertical L9
  constraint midpoint L4 L6.start
  constraint horizontal L10
  constraint vertical L11
  constraint horizontal L12
  constraint vertical L13
  constraint horizontal L14
  constraint vertical L15
  constraint horizontal L16
  constraint vertical L17
  constraint horizontal L18
  constraint vertical L19
  constraint coincident L5 L16.start
  measures "d142" distance of L6.start L8.end
  measures "d143" distance of L6.start L10.end
  measures "d149" distance of L16.start L18.end
extrude "Extrude18" cut sketch "Sketch19" against normal blind 3 contours L4 L6 L7 L8 L9 L11 L15 | L4 L9 L10 L11 L12 L13 L14 L15 bodies 15
sketch "Sketch20" plane through (111.5, 0, 0) normal (1, 0, 0) x (0, 1, 0)
  line L0 (10, 40) -> (20, 40)
  line L1 (20, 40) -> (20, 43)
  line L2 (20, 43) -> (10, 43)
  line L3 (10, 43) -> (10, 40)
  line L4 (10, 40) -> (20, 40)
  line L5 (20, 40) -> (20, 41.5)
  line L6 (20, 41.5) -> (10, 41.5)
  line L7 (10, 41.5) -> (10, 40)
  dimension "d146" = 1.5
  constraint horizontal L4
  constraint vertical L5
  constraint horizontal L6
  constraint vertical L7
  constraint coincident L0.start L3.end
  measures "d146" distance of L0.start L6.end
extrude "Extrude19" cut sketch "Sketch20" against normal blind 3 contours L0 L1 L3 L4 L5 L6 L7 bodies 16
move_body "Move46" bodies 16 to x (1, 0, 0) y (0, 1, 0) z (0, 0, 1) at (0, 0, -3)
extrude "Extrude20" cut sketch "Sketch19" against normal blind 3 contours L5 L16 L17 L18 L19 bodies 15
move_body "Move47" bodies 16 to x (1, 0, 0) y (0, -1, 0) z (0, 0, -1) at (0, 30, 30)
move_body "Move48" bodies 10 9 13 14 to x (1, 0, 0) y (0, 1, 0) z (0, 0, 1) at (-1, 0, 4.9)
move_body "Move49" bodies 5 6 to x (1, 0, 0) y (0, 1, 0) z (0, 0, 1) at (0, 1, 5)
move_body "Move50" bodies 6 to x (1, 0, 0) y (0, 1, 0) z (0, 0, 1) at (0, -2, -0.2)
sketch "Sketch21" plane through (74.5, 0, 0) normal (1, 0, 0) x (0, 1, 0)
  line L0 (5, -7) -> (-23, -7)
  line L1 (-23, -7) -> (-23, -10)
  line L2 (-23, -10) -> (5, -10)
  line L3 (5, -10) -> (5, -7)
  line L4 (-30, 35) -> (60, 35)
  line L5 (60, 35) -> (60, -5)
  line L6 (60, -5) -> (-30, -5)
  line L7 (-30, -5) -> (-30, 35)
  circle A0 centre (-7.9, 15.1) radius 6.1
  circle A1 centre (37.9049, 15.1047) radius 6.1
  circle A2 centre (-2.0555, 15.1538) radius 2
  circle A3 centre (32.0504, 15.0437) radius 2
  line L8 (-18.9, 21.2) -> (-14.1, 21.2)
  line L9 (-14.1, 21.2) -> (-14.1, 9)
  line L10 (-14.1, 9) -> (-18.9, 9)
  line L11 (-18.9, 9) -> (-18.9, 21.2)
  line L12 (8.9, 9) -> (13.7, 9)
  line L13 (13.7, 9) -> (13.7, 21.2)
  line L14 (13.7, 21.2) -> (8.9, 21.2)
  line L15 (8.9, 21.2) -> (8.9, 9)
  line L16 (16.3, 21.2) -> (21.1, 21.2)
  line L17 (21.1, 21.2) -> (21.1, 9)
  line L18 (21.1, 9) -> (16.3, 9)
  line L19 (16.3, 9) -> (16.3, 21.2)
  line L20 (44.1, 9) -> (48.9, 9)
  line L21 (48.9, 9) -> (48.9, 21.2)
  line L22 (48.9, 21.2) -> (44.1, 21.2)
  line L23 (44.1, 21.2) -> (44.1, 9)
  circle A4 centre (-17, 15) radius 1
  circle A5 centre (12, 15) radius 1
  circle A6 centre (18, 15) radius 1
  circle A7 centre (47, 15) radius 1
  dimension "d152" = 90
  dimension "d153" = 40
  dimension "d154" = 12.2
  dimension "d155" = 12.2
  dimension "d156" = 4
  dimension "d157" = 4
  constraint horizontal L4
  constraint vertical L5
  constraint horizontal L6
  constraint vertical L7
  constraint horizontal L8
  constraint vertical L9
  constraint horizontal L10
  constraint vertical L11
  constraint horizontal L12
  constraint vertical L13
  constraint horizontal L14
  constraint vertical L15
  constraint horizontal L16
  constraint vertical L17
  constraint horizontal L18
  constraint vertical L19
  constraint horizontal L20
  constraint vertical L21
  constraint horizontal L22
  constraint vertical L23
  measures "d152" distance of L4.start L4.end
  measures "d153" distance of L4.start L6.end
  measures "d154" diameter of A0
  measures "d155" diameter of A1
  measures "d156" diameter of A2
  measures "d157" diameter of A3
extrude "Extrude21" add sketch "Sketch21" against normal blind 3 separate body contours L4 L5 L6 L7 makes body 17
fillet "Fillet14" radius 20 4 edges at (73, -30, 35) (73, -30, -5) (73, 60, 35) (73, 60, -5) on bodies 17
extrude "Extrude22" add sketch "Sketch21" against normal blind 6 contours L8 L9 L10 L11 | L12 L13 L14 L15 | L16 L17 L18 L19 | L20 L21 L22 L23 bodies 17
sketch "Sketch22" plane through (71.5, 0, 0) normal (-1, 0, 0) x (0, -1, 0)
  arc A0 (-40, 35) -> (-40, -5) centre (-40, 15) ccw
  line L0 (-40, -5) -> (10, -5)
  arc A1 (10, -5) -> (10, 35) centre (10, 15) ccw
  line L1 (10, 35) -> (-40, 35)
  line L2 (-8.9, 21.2) -> (-8.9, 9)
  line L3 (-8.9, 9) -> (-13.7, 9)
  line L4 (-13.7, 9) -> (-13.7, 21.2)
  line L5 (-13.7, 21.2) -> (-8.9, 21.2)
  line L6 (18.9, 9) -> (14.1, 9)
  line L7 (14.1, 9) -> (14.1, 21.2)
  line L8 (14.1, 21.2) -> (18.9, 21.2)
  line L9 (18.9, 21.2) -> (18.9, 9)
  line L10 (-16.3, 9) -> (-21.1, 9)
  line L11 (-21.1, 9) -> (-21.1, 21.2)
  line L12 (-21.1, 21.2) -> (-16.3, 21.2)
  line L13 (-16.3, 21.2) -> (-16.3, 9)
  line L14 (-44.1, 21.2) -> (-44.1, 9)
  line L15 (-44.1, 9) -> (-48.9, 9)
  line L16 (-48.9, 9) -> (-48.9, 21.2)
  line L17 (-48.9, 21.2) -> (-44.1, 21.2)
  arc A2 (2.1553, 17.1513) -> (2.1185, 13.1548) centre (2.0555, 15.1538) ccw
  arc A3 (2.1185, 13.1548) -> (2.1553, 17.1513) centre (7.9, 15.1) ccw
  arc A4 (-32.1209, 17.0424) -> (-32.1625, 13.0468) centre (-37.9049, 15.1047) ccw
  arc A5 (-32.1625, 13.0468) -> (-32.1209, 17.0424) centre (-32.0504, 15.0437) ccw
  line L18 (23, -2) -> (-53, -2)
  line L19 (-53, -2) -> (-53, -5)
  line L20 (-53, -5) -> (23, -5)
  line L21 (23, -5) -> (23, -2)
  line L22 (10, -5) -> (5, -5)
  line L23 (-34.949, -5) -> (-40, -5)
  line L24 (-34.949, -5) -> (-39.949, -5)
  line L25 (-39.949, -5) -> (-39.949, 3)
  line L26 (-39.949, 3) -> (-34.949, 3)
  line L27 (-34.949, 3) -> (-34.949, -5)
  line L28 (10, -5) -> (5, -5)
  line L29 (5, -5) -> (5, -2)
  line L30 (5, -2) -> (10, -2)
  line L31 (10, -2) -> (10, -5)
  line L32 (-15, 35) -> (-10, 35)
  line L33 (-10, 35) -> (-10, 33.5)
  line L34 (-10, 33.5) -> (-15, 33.5)
  line L35 (-15, 33.5) -> (-15, 35)
  line L36 (-15, 35) -> (-20, 35)
  line L37 (-20, 35) -> (-20, 33.5)
  line L38 (-20, 33.5) -> (-15, 33.5)
  line L39 (-15, 33.5) -> (-15, 35)
  dimension "d168" = 5
  dimension "d170" = 5
  dimension "d176" = 5
  dimension "d177" = 1.5
  dimension "d178" = 5
  constraint horizontal L18
  constraint vertical L19
  constraint horizontal L20
  constraint vertical L21
  constraint horizontal L22
  constraint coincident L0 A1.start
  constraint coincident L20 L0.end
  constraint horizontal L23
  constraint coincident L20 L23.start
  constraint horizontal L24
  constraint vertical L25
  constraint horizontal L26
  constraint vertical L27
  constraint horizontal L28
  constraint vertical L29
  constraint horizontal L30
  constraint vertical L31
  constraint coincident L18 L29.end
  constraint horizontal L32
  constraint vertical L33
  constraint horizontal L34
  constraint vertical L35
  constraint midpoint L1 L32.start
  constraint horizontal L36
  constraint vertical L37
  constraint horizontal L38
  constraint vertical L39
  measures "d168" distance of L0.end L22.end
  measures "d170" distance of L23.start L24.end
  measures "d176" distance of L32.start L32.end
  measures "d177" distance of L32.start L34.end
  measures "d178" distance of L32.start L36.end
extrude "Extrude24" cut sketch "Sketch22" against normal blind 3 contours A0 L0 L18 L20 L23 L25 | L0 L18 L20 L27 L29 | A1 L18 L31 | A1 L18 L20 L21 bodies 17
sketch "Sketch23" plane through (74.5, 0, 0) normal (1, 0, 0) x (0, 1, 0)
  line L0 (5, -7) -> (-23, -7)
  line L1 (-23, -7) -> (-23, -10)
  line L2 (-23, -10) -> (5, -10)
  line L3 (5, -10) -> (5, -7)
  line L4 (-10, -10) -> (-5, -10)
  line L5 (-5, -10) -> (-5, -7)
  line L6 (-5, -7) -> (-10, -7)
  line L7 (-10, -7) -> (-10, -10)
  line L8 (35, 0) -> (40, 0)
  line L9 (40, 0) -> (40, 3)
  line L10 (40, 3) -> (35, 3)
  line L11 (35, 3) -> (35, 0)
  dimension "d173" = 5
  constraint horizontal L4
  constraint vertical L5
  constraint horizontal L6
  constraint vertical L7
  constraint coincident L2 L4.start
  constraint horizontal L8
  constraint vertical L9
  constraint horizontal L10
  constraint vertical L11
  measures "d173" distance of L4.start L4.end
extrude "Extrude25" cut sketch "Sketch23" against normal blind 3 contours L0 L2 L4 L5 L6 L7 | L8 L9 L10 L11 bodies 16
extrude "Extrude26" cut sketch "Sketch22" against normal blind 3 contours L1 L35 L36 L37 L38 L39 | L1 L32 L33 L34 L35 L39 bodies 17
sketch "Sketch24" plane through (0, 0, 35) normal (0, 0, 1) x (-1, 0, 0)
  line L0 (-74.5, -10) -> (-71.5, -10)
  line L1 (-71.5, -10) -> (-71.5, 10)
  line L2 (-74.5, 10) -> (-74.5, -10)
  line L3 (-155, -5) -> (-115, -5)
  line L4 (-115, -5) -> (-115, -25)
  line L5 (-115, -25) -> (-155, -25)
  line L6 (-155, -25) -> (-155, -5)
  line L7 (-115, -25) -> (-118, -25)
  line L8 (-118, -25) -> (-118, -20)
  line L9 (-118, -20) -> (-115, -20)
  line L10 (-115, -20) -> (-115, -25)
  line L11 (-115, -5) -> (-118, -5)
  line L12 (-118, -5) -> (-118, -10)
  line L13 (-118, -10) -> (-115, -10)
  line L14 (-115, -10) -> (-115, -5)
  line L15 (-155, -25) -> (-152, -25)
  line L16 (-152, -25) -> (-152, -20)
  line L17 (-152, -20) -> (-155, -20)
  line L18 (-155, -20) -> (-155, -25)
  line L19 (-155, -5) -> (-152, -5)
  line L20 (-152, -5) -> (-152, -10)
  line L21 (-152, -10) -> (-155, -10)
  line L22 (-155, -10) -> (-155, -5)
  line L23 (-115, -20) -> (-118, -20)
  line L24 (-118, -20) -> (-118, -10)
  line L25 (-118, -10) -> (-115, -10)
  line L26 (-115, -10) -> (-115, -20)
  line L27 (-152, -20) -> (-155, -20)
  line L28 (-155, -20) -> (-155, -10)
  line L29 (-155, -10) -> (-152, -10)
  line L30 (-152, -10) -> (-152, -20)
  line L31 (-71.5, 10) -> (-74.5, 10)
  dimension "d181" = 40
  dimension "d182" = 20
  constraint horizontal L3
  constraint vertical L4
  constraint horizontal L5
  constraint vertical L6
  constraint horizontal L7
  constraint vertical L8
  constraint horizontal L9
  constraint vertical L10
  constraint horizontal L11
  constraint vertical L12
  constraint horizontal L13
  constraint vertical L14
  constraint horizontal L15
  constraint vertical L16
  constraint horizontal L17
  constraint vertical L18
  constraint horizontal L19
  constraint vertical L20
  constraint horizontal L21
  constraint vertical L22
  constraint horizontal L23
  constraint vertical L24
  constraint horizontal L25
  constraint vertical L26
  constraint horizontal L27
  constraint vertical L28
  constraint horizontal L29
  constraint vertical L30
  measures "d181" distance of L3.start L3.end
  measures "d182" distance of L3.start L5.end
extrude "Extrude27" add sketch "Sketch24" against normal blind 3 separate body contours L3 L5 L8 L12 L16 L20 L24 L30 makes body 18
extrude "Extrude28" add sketch "Sketch24" against normal blind 1.5 contours L6 L17 L21 L27 L28 L29 L30 | L4 L9 L13 L23 L24 L25 L26 bodies 18
move_body "Move51" bodies 18 to x (1, 0, 0) y (0, 1, 0) z (0, 0, 1) at (-43.5, 0, 0)
copy_body "CopyPasteBodies7" bodies 15 makes body 19
move_body "Move52" bodies 19 to x (-1, 0, 0) y (0, -1, 0) z (0, 0, 1) at (39, 30, 0)
sketch "Sketch25" plane through (-72.5, 0, 0) normal (-1, 0, 0) x (0, -1, 0)
  line L0 (-10, -7) -> (-20, -7)
  line L1 (-20, -7) -> (-20, -10)
  line L2 (-20, -10) -> (-10, -10)
  line L3 (-10, -10) -> (-10, -7)
  line L4 (-20, -7) -> (-10, -7)
  line L5 (-10, -7) -> (-10, -8.5)
  line L6 (-10, -8.5) -> (-20, -8.5)
  line L7 (-20, -8.5) -> (-20, -7)
  constraint horizontal L4
  constraint vertical L5
  constraint horizontal L6
  constraint vertical L7
  constraint midpoint L3 L5.end
  constraint coincident L0.end L1.start
extrude "Extrude29" cut sketch "Sketch25" against normal blind 3 contours L0 L1 L3 L4 L5 L6 L7 bodies 16
copy_body "CopyPasteBodies8" bodies 17 makes body 20
move_body "Move53" bodies 20 to x (-1, 0, 0) y (0, -1, 0) z (0, 0, 1) at (39, 30, 0)
sketch "Sketch26" plane through (-35.5, 0, 0) normal (-1, 0, 0) x (0, -1, 0)
  line L0 (-25, -7) -> (-53, -7)
  line L1 (-53, -7) -> (-53, -10)
  line L2 (-53, -10) -> (-25, -10)
  line L3 (-25, -10) -> (-25, -7)
  line L4 (-40, -10) -> (-35, -10)
  line L5 (-35, -10) -> (-35, -7)
  line L6 (-35, -7) -> (-40, -7)
  line L7 (-40, -7) -> (-40, -10)
  line L8 (5, 0) -> (10, 0)
  line L9 (10, 0) -> (10, 3)
  line L10 (10, 3) -> (5, 3)
  line L11 (5, 3) -> (5, 0)
  dimension "d189" = 5
  constraint horizontal L4
  constraint vertical L5
  constraint horizontal L6
  constraint vertical L7
  constraint coincident L2 L4.start
  constraint horizontal L8
  constraint vertical L9
  constraint horizontal L10
  constraint vertical L11
  measures "d189" distance of L4.start L4.end
extrude "Extrude30" cut sketch "Sketch26" against normal blind 3 contours L0 L2 L4 L5 L6 L7 | L8 L9 L10 L11 bodies 16
copy_body "CopyPasteBodies9" bodies 18 makes body 21
move_body "Move54" bodies 21 to x (1, 0, 0) y (0, 1, 0) z (0, 0, 1) at (-144, 0, 0)
move_body "Move55" bodies 4 to x (1, 0, 0) y (0, 1, 0) z (0, 0, 1) at (-1.5, 1, 4.8)
move_body "Move56" bodies 1 to x (1, 0, 0) y (0, 1, 0) z (0, 0, 1) at (-1.5, -1, 5)
move_body "Move57" bodies 11 to x (1, 0, 0) y (0, 1, 0) z (0, 0, 1) at (0, 0, 5)
move_body "Move58" bodies 12 to x (1, 0, 0) y (0, 1, 0) z (0, 0, 1) at (0, 0, 5)
move_body "Move59" bodies 8 to x (1, 0, 0) y (0, 1, 0) z (0, 0, 1) at (0, 0, 5)
move_body "Move60" bodies 7 to x (1, 0, 0) y (0, 1, 0) z (0, 0, 1) at (0, 0, 5)
move_body "Move61" bodies 2 to x (1, 0, 0) y (0, 1, 0) z (0, 0, 1) at (-0.8, 0, -1)